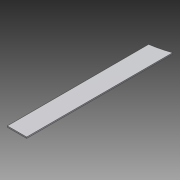
# Autodesk Inventor part: Hopper Teflon Strip P2
Saved by Autodesk Inventor 2014 SP1 (Build 180222100, 222)
## iProperties
Created: 2013-12-17
Part Number: Hopper Teflon Strip P2
Material: Generic
Document SubType Name: Modeling
Designer: Moses
Density: 1 g/cm^3
Appearance: White
Mass: 7.60437 g
Surface Area: 102.623 cm^2
Volume: 7.60437 cm^3
Author: Moses
Autodesk Inventor part; units mm, degrees
ref_plane "YZ Plane" through (0, 0, 0) normal (1, 0, 0) x (0, 1, 0)
ref_plane "XZ Plane" through (0, 0, 0) normal (0, 1, 0) x (-1, 0, 0)
ref_plane "XY Plane" through (0, 0, 0) normal (0, 0, 1) x (1, 0, 0)
sketch "Sketch1" plane through (0, 0, 0) normal (0, 1, 0) x (-1, 0, 0)
  line L0 (0, 0) -> (0, 330.2) construction
  line L1 (0, 330.2) -> (330.2, 330.2) construction
  line L2 (330.2, 330.2) -> (330.2, 0) construction
  line L3 (330.2, 0) -> (0, 0) construction
  circle A0 centre (146.05, 0) radius 146.05 construction
  line L4 (98.425, 138.0669) -> (98.425, 330.2)
  line L5 (98.425, 330.2) -> (123.825, 330.2)
  line L6 (123.825, 330.2) -> (123.825, 144.3491)
  arc A1 (123.825, 144.3491) -> (98.425, 138.0669) centre (146.05, 0) ccw
  dimension "d0" = 292.1
  dimension "d1" = 330.2
  dimension "d2" = 330.2
  dimension "d4" = 25.4
  dimension "d8" = 98.425
  constraints: 14 end point, 5 point on circle, 4 vertical, 2 centre point, 2 horizontal, 2 point on line, 1 concentric, 1 tangent
  measures "d0" diameter of A0
  measures "d1" distance of L0.start L0.end
  measures "d2" distance of L0.end L1.end
  measures "d4" distance between parallel lines of L6 L4
  measures "d8" distance between parallel lines of L4 L0
extrude "Extrusion1" add sketch "Sketch1" along normal blind 1.5875
body "Solid1"
